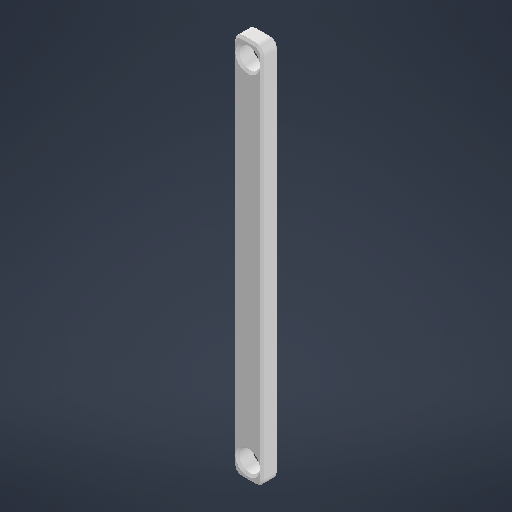
# Autodesk Inventor part: Spacer
Saved by Autodesk Inventor 2026.3 (Build 303398000, 398)
## iProperties
Created: 2026-05-02
Part Number: Spacer
Material: Generic
Document SubType Name: Modeling
Designer: frede
Density: 1 g/cm^3
Appearance: Default
Author: frede
Autodesk Inventor part; units mm, degrees
ref_plane "YZ Plane" through (0, 0, 0) normal (1, 0, 0) x (0, 1, 0)
ref_plane "XZ Plane" through (0, 0, 0) normal (0, 1, 0) x (-1, 0, 0)
ref_plane "XY Plane" through (0, 0, 0) normal (0, 0, 1) x (1, 0, 0)
sketch "Sketch1" plane through (0, 0, 0) normal (0, 0, 1) x (1, 0, 0)
  line L0 (-2, 0) -> (-5, 0)
  line L1 (-7, 2) -> (-7, 90)
  line L2 (-5, 92) -> (-2, 92)
  line L3 (0, 90) -> (0, 2)
  circle A0 centre (-3.5, 4) radius 2.5
  circle A1 centre (-3.5, 88) radius 2.5
  arc A2 (-5, 92) -> (-7, 90) centre (-5, 90) ccw
  arc A3 (0, 90) -> (-2, 92) centre (-2, 90) ccw
  arc A4 (-2, 0) -> (0, 2) centre (-2, 2) ccw
  arc A5 (-7, 2) -> (-5, 0) centre (-5, 2) ccw
  point P0 (0, 0)
  point P1 (-7, 92)
  point P2 (-7, 0)
  point P3 (0, 92)
  point P4 (-3.5, 92)
  dimension "d0" = 7
  dimension "d1" = 92
  dimension "d2" = 5
  dimension "d3" = 5
  dimension "d4" = 84
  dimension "d5" = 4
  dimension "d6" = 2
  constraints: 8 end point, 8 point on circle, 8 point on line, 8 tangent, 6 centre point, 3 equal radius, 2 parallel, 1 horizontal, 1 midpoint, 1 perpendicular
  measures "d0" distance of point (-7, 92) point (0, 92)
  measures "d1" distance of point (-7, 0) point (-7, 92)
  measures "d2" diameter of A0
  measures "d3" diameter of A1
  measures "d4" distance of A0.centre A1.centre
  measures "d5" distance of point (-3.5, 92) A1.centre
  measures "d6" radius of A2
extrude "Extrusion1" add sketch "Sketch1" along normal blind 4
chamfer "Chamfer1" distance 0.5 angle 45 20 edges at (-6, 88, 4) (-6, 88, 0) (-3.5, 92, 0) (-6.4142, 91.4142, 0) (-7, 46, 0) (-6.4142, 0.5858, 0) (-3.5, 0, 0) (-0.5858, 0.5858, 0) (0, 46, 0) (-0.5858, 91.4142, 0) (-3.5, 92, 4) (-6.4142, 91.4142, 4) (-7, 46, 4) (-6.4142, 0.5858, 4) (-3.5, 0, 4) (-0.5858, 0.5858, 4) (0, 46, 4) (-0.5858, 91.4142, 4) (-6, 4, 4) (-6, 4, 0)
equation "\"d5\" = -0.5 * d4 + 0.5 * d1"
body "Solid1"
